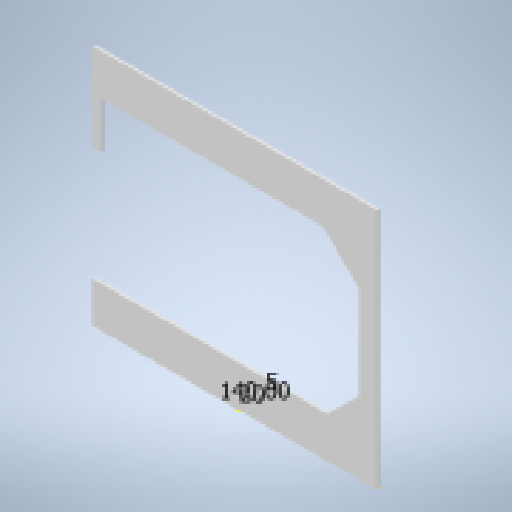
# Autodesk Inventor part: sensor board
Saved by Autodesk Inventor 2025 (Build 290162000, 162)
## iProperties
Created: 2026-07-27
Part Number: sensor board
Material: Типовые
Document SubType Name: Modeling
Designer: garin
Density: 1 g/cm^3
Appearance: По умолчанию
Author: garin
Autodesk Inventor part; units mm, degrees
ref_plane "YZ Plane" through (0, 0, 0) normal (1, 0, 0) x (0, 1, 0)
ref_plane "XZ Plane" through (0, 0, 0) normal (0, 1, 0) x (-1, 0, 0)
ref_plane "XY Plane" through (0, 0, 0) normal (0, 0, 1) x (1, 0, 0)
sketch "Эскиз1" plane through (0, 0, 0) normal (0, 0, 1) x (1, 0, 0)
  line L0 (0, 0) -> (-80.25, 0) construction
  line L1 (-80.25, 0) -> (-80.25, -18.086) construction
  line L2 (-80.25, -18.086) -> (0, -18.086) construction
  line L3 (0, -18.086) -> (0, 0) construction
  line L4 (-80.25, -18.086) -> (-80.25, -40.587) construction
  line L5 (-80.25, -18.086) -> (-57.749, -18.086) construction
  line L6 (-80.25, -40.587) -> (76.75, -40.587)
  line L7 (76.75, -40.587) -> (76.75, 92.813)
  line L8 (76.75, 92.813) -> (-80.25, 92.813)
  line L9 (-80.25, 92.813) -> (-80.25, -40.587)
  line L10 (-80.25, -40.587) -> (76.75, -40.587)
  line L11 (76.75, -40.587) -> (76.75, -18.087)
  line L12 (76.75, -18.087) -> (-80.25, -18.087)
  line L13 (-80.25, -18.087) -> (-80.25, -40.587)
  line L14 (76.75, 92.813) -> (-80.25, 92.813)
  line L15 (-80.25, 92.813) -> (-80.25, 70.313)
  line L16 (-80.25, 70.313) -> (76.75, 70.313)
  line L17 (76.75, 70.313) -> (76.75, 92.813)
  line L18 (-80.25, -40.587) -> (-75.25, -40.587)
  line L19 (-75.25, -40.587) -> (-75.25, 90.413)
  line L20 (-75.25, 90.413) -> (-80.25, 90.413)
  line L21 (-80.25, 90.413) -> (-80.25, -40.587)
  line L22 (76.75, -40.587) -> (66.75, -40.587)
  line L23 (66.75, -40.587) -> (66.75, 90.413)
  line L24 (66.75, 90.413) -> (76.75, 90.413)
  line L25 (76.75, 90.413) -> (76.75, -40.587)
  line L26 (76.75, -40.587) -> (41.75, -40.587)
  line L27 (41.75, -40.587) -> (41.75, -20.587)
  line L28 (41.75, -40.587) -> (61.75, -40.587) construction
  line L29 (76.75, 24.913) -> (-80.25, 24.913)
  line L30 (41.75, 90.413) -> (41.75, 70.413)
  line L31 (66.75, 70.313) -> (66.75, 50.313)
  line L32 (66.75, 50.313) -> (46.75, 70.313)
  line L33 (66.75, 50.313) -> (95.0343, 50.313) construction
  line L34 (66.75, -0.487) -> (46.75, -20.487)
  line L35 (-75.25, 24.913) -> (-80.25, 24.913)
  line L36 (-80.25, 24.913) -> (-80.25, 44.913)
  line L37 (-80.25, 44.913) -> (-75.25, 44.913)
  line L38 (-75.25, 44.913) -> (-75.25, 24.913)
  point P0 (-75.25, -18.087)
  point P1 (-75.25, 70.313)
  point P2 (71.75, 70.413)
  point P3 (66.75, -18.087)
  point P4 (66.75, -0.487)
  point P5 (49.15, -18.087)
  point P6 (-80.25, 44.913)
  point P7 (-75.25, 44.913)
  dimension "d0" = 80.25
  dimension "d1" = 18.086
  dimension "d2" = 22.501
  dimension "d3" = 90
  dimension "d4" = 157
  dimension "d5" = 133.4
  dimension "d6" = 157
  dimension "d7" = 22.5
  dimension "d8" = 157
  dimension "d9" = 22.5
  dimension "d10" = 5
  dimension "d11" = 131
  dimension "d12" = 10
  dimension "d13" = 131
  dimension "d16" = 35
  dimension "d17" = 20
  dimension "d18" = 90
  dimension "d19" = 20
  dimension "d20" = 135
  dimension "d21" = 20
  constraints: 78 end point, 15 parallel, 10 horizontal, 7 perpendicular, 7 point on line, 4 symmetric about line, 3 equal length, 3 midpoint, 1 vertical
  measures "d0" distance of L2.end L1.end
  measures "d1" distance of L1.end L0.end
  measures "d2" distance of L1.end L4.end
  measures "d3" angle of L4 L5
  measures "d4" distance of L8.end L7.end
  measures "d5" distance of L7.end L6.end
  measures "d6" distance of L12.end L11.end
  measures "d7" distance of L11.end L10.end
  measures "d8" distance of L16.end L15.end
  measures "d9" distance of L15.end L14.end
  measures "d10" distance of L20.end L19.end
  measures "d11" distance of L19.end L18.end
  measures "d12" distance of L23.end L24.end
  measures "d13" distance of L22.end L23.end
  measures "d16" distance of L10.end L26.end
  measures "d17" distance of L26.end L27.end
  measures "d18" angle of L28 L27
  measures "d19" distance of L31.start L31.end
  measures "d20" angle of L33 L32
  measures "d21" distance of L35.end L36.end
extrude "Выдавливание1" add sketch "Эскиз1" along normal blind 1.5 contours L9 L12 L19 L6 | L19 L12 L23 L6 | L23 L12 L7 L6 | L34 L23 L12 | L9 L16 L19 L37 | L23 L29 L7 L12 | L23 L16 L7 L29 | L9 L20 L19 L16 | L19 L20 L9 L8 L7 L24 L23 L16 | L32 L16 L23 | L23 L24 L7 L16
sketch "Эскиз2" plane through (-80.25, -40.587, 0) normal (0, -1, 0) x (1, 0, 0)
  line L0 (129.4, 0) -> (0, 0) projected
  line L1 (157, 0) -> (0, 0) projected
  line L2 (0, 0) -> (157, 0)
  line L3 (157, 0) -> (78.5, 0)
  line L4 (78.5, 0) -> (78.5, -20)
  line L5 (78.5, -20) -> (73.5, -20)
  line L6 (73.5, -20) -> (49.6649, 0)
  line L7 (78.5, -20) -> (83.5, -20)
  line L8 (83.5, -20) -> (107.3351, 0)
  point P0 (80.25, 0)
  dimension "d22" = 20
  dimension "d24" = 5
  dimension "d25" = 140
  constraints: 14 end point, 2 symmetric about line, 1 collinear, 1 horizontal, 1 midpoint, 1 perpendicular, 1 point on line
  measures "d22" distance of L3.end L4.end
  measures "d24" distance of L4.end L5.end
  measures "d25" angle of L5 L6
